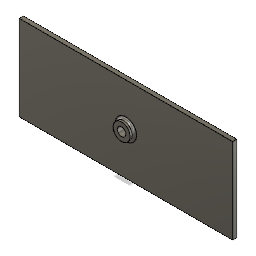
Table_17p1_Problem_14 (Autodesk Fusion 360 design; units mm, degrees)
Autodesk Fusion 360 part; units mm, degrees
sketch "Sketch1" plane through (0, 0, 0) normal (0, 0, 1) x (1, 0, 0)
  line L0 (-250, 100) -> (250, 100)
  line L1 (250, 100) -> (250, -100)
  line L2 (250, -100) -> (-250, -100)
  line L3 (-250, -100) -> (-250, 100)
  line L4 (0, 100) -> (0, -100) construction
  line L5 (-250, 0) -> (250, 0) construction
  circle A0 centre (0, 0) radius 20
  circle A1 centre (0, 0) radius 10
  dimension "Total_Height" = 200
  dimension "Total_Width" = 500
  dimension "Inner_Radius" = 10
  dimension "Outer_Radius" = 20
  constraint horizontal L0
  constraint vertical L1
  constraint horizontal L2
  constraint vertical L3
  constraint coincident A0.centre A1.centre
  constraint midpoint L0 L4.start
  constraint midpoint L2 L4.end
  constraint midpoint L3 L5.start
  constraint midpoint L1 L5.end
  constraint coincident A0.centre L5
  constraint coincident A0.centre L4
  constraint concentric A0 A1
  measures "Total_Height" distance of L0.start L2.end
  measures "Total_Width" distance of L0.start L0.end
  measures "Inner_Radius" radius of A1
  measures "Outer_Radius" radius of A0
extrude "Extrude1" add sketch "Sketch1" along normal mid plane 10 contours L0 L1 L2 L3
extrude "Extrude2" add sketch "Sketch1" along normal mid plane 30 contours A0
fillet "Fillet1" radius 5 2 edges at (-18.6465, 7.2323, 5) (-18.6465, -7.2323, -5)
equation "Plate_Thickness = 1 cm"
equation "Shoulder_Thickness = 3 cm"
equation "Fillet_Radius = 0.5 cm"
